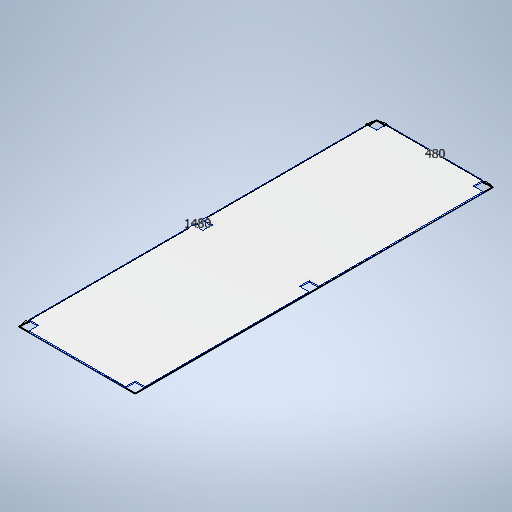
# Autodesk Inventor part: cupboard floor
Saved by Autodesk Inventor 2025 (Build 290162010, 162A)
## iProperties
Created: 2024-06-14
Part Number: cupboard floor
Material: Aluminum 6061
Document SubType Name: Modeling
Designer: Alan Thomas
Mass: 9460.8 g
Surface Area: 14220 cm^2
Volume: 3504 cm^3
Density: 2.7 g/cm^3
Appearance: Aluminum - Flat
Author: Alan Thomas
Autodesk Inventor part; units mm, degrees
ref_plane "YZ Plane" through (0, 0, 0) normal (1, 0, 0) x (0, 1, 0)
ref_plane "XZ Plane" through (0, 0, 0) normal (0, 1, 0) x (-1, 0, 0)
ref_plane "XY Plane" through (0, 0, 0) normal (0, 0, 1) x (1, 0, 0)
sketch "Sketch1" plane through (0, 0, 0) normal (0, 1, 0) x (-1, 0, 0)
  line L0 (0, 0) -> (480, 0)
  line L1 (480, 0) -> (480, -1480)
  line L2 (480, -1480) -> (0, -1480)
  line L3 (0, -1480) -> (0, 0)
  dimension "d0" = 480
  dimension "d1" = 1480
  constraints: 8 end point, 2 parallel, 1 horizontal, 1 perpendicular
  measures "d0" distance of L1.end L2.end
  measures "d1" distance of L0.end L1.end
extrude "Extrusion1" add sketch "Sketch1" along normal blind 5
sketch "Sketch2" plane through (0, 5, 0) normal (0, 1, 0) x (1, 0, 0)
  line L0 (-480, 1480) -> (-480, 0) projected
  line L1 (-480, 0) -> (-440, 0)
  line L2 (-440, 0) -> (-440, 40)
  line L3 (-440, 40) -> (-480, 40)
  line L4 (-480, 40) -> (-480, 0)
  point P0 (0, 0)
  dimension "d4" = 40
  dimension "d5" = 40
  constraints: 8 end point, 2 parallel, 1 horizontal, 1 perpendicular
  measures "d4" distance of L3.end L2.end
  measures "d5" distance of L2.end L1.end
extrude "Extrusion2" cut sketch "Sketch2" against normal blind 10
sketch "Sketch3" plane through (0, 5, 0) normal (0, 1, 0) x (1, 0, 0)
  line L0 (-440, 0) -> (0, 0) projected
  line L1 (0, 0) -> (-40, 0)
  line L2 (-40, 0) -> (-40, 40)
  line L3 (-40, 40) -> (0, 40)
  line L4 (0, 40) -> (0, 0)
  line L5 (0, 1480) -> (-480, 1480) projected
  line L6 (0, 1480) -> (-40, 1480)
  line L7 (-40, 1480) -> (-40, 1440)
  line L8 (-40, 1440) -> (0, 1440)
  line L9 (0, 1440) -> (0, 1480)
  line L10 (-480, 1480) -> (-440, 1480)
  line L11 (-440, 1480) -> (-440, 1440)
  line L12 (-440, 1440) -> (-480, 1440)
  line L13 (-480, 1440) -> (-480, 1480)
  dimension "d8" = 40
  dimension "d9" = 40
  dimension "d10" = 40
  dimension "d11" = 40
  dimension "d12" = 40
  dimension "d13" = 40
  constraints: 24 end point, 6 parallel, 3 horizontal, 3 perpendicular
  measures "d8" distance of L2.end L3.end
  measures "d9" distance of L1.end L2.end
  measures "d10" distance of L8.end L7.end
  measures "d11" distance of L7.end L6.end
  measures "d12" distance of L11.end L12.end
  measures "d13" distance of L10.end L11.end
extrude "Extrusion3" cut sketch "Sketch3" against normal blind 10
sketch "Sketch7" plane through (0, 5, 0) normal (0, 1, 0) x (1, 0, 0)
  line L0 (0, 40) -> (0, 1440) projected
  line L1 (0, 720) -> (-40, 720)
  line L2 (-40, 720) -> (-40, 760)
  line L3 (-40, 760) -> (0, 760)
  line L4 (0, 760) -> (0, 720)
  line L5 (-480, 1440) -> (-480, 40) projected
  line L6 (-480, 720) -> (-440, 720)
  line L7 (-440, 720) -> (-440, 760)
  line L8 (-440, 760) -> (-480, 760)
  line L9 (-480, 760) -> (-480, 720)
  point P0 (0, 0)
  point P1 (0, 760)
  dimension "d29" = 40
  dimension "d30" = 40
  dimension "d31" = 40
  dimension "d32" = 40
  constraints: 16 end point, 4 parallel, 3 point on line, 2 horizontal, 2 perpendicular
  measures "d29" distance of L2.end L3.end
  measures "d30" distance of L1.end L2.end
  measures "d31" distance of L8.end L7.end
  measures "d32" distance of L7.end L6.end
extrude "Extrusion7" cut sketch "Sketch7" against normal blind 10
body "Solid1"
